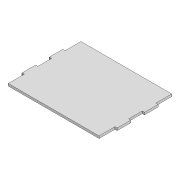
# Autodesk Inventor part: Tapa diagonal
Saved by Autodesk Inventor 2022 (Build 260153000, 153)
## iProperties
Created: 2022-06-16
Part Number: Tapa diagonal
Material: Generic
Document SubType Name: Modeling
Designer: ADMIN
Density: 1 g/cm^3
Appearance: Default
Author: ADMIN
Autodesk Inventor part; units mm, degrees
ref_plane "YZ Plane" through (0, 0, 0) normal (1, 0, 0) x (0, 1, 0)
ref_plane "XZ Plane" through (0, 0, 0) normal (0, 1, 0) x (-1, 0, 0)
ref_plane "XY Plane" through (0, 0, 0) normal (0, 0, 1) x (1, 0, 0)
sketch "Sketch1" plane through (0, 0, 0) normal (0, 1, 0) x (-1, 0, 0)
  line L0 (-88.7139, 28.3135) -> (111.2861, 28.3135)
  line L1 (111.2861, 28.3135) -> (111.2861, -131.6865)
  line L2 (111.2861, -131.6865) -> (-88.7139, -131.6865)
  line L3 (-88.7139, -131.6865) -> (-88.7139, 28.3135)
  line L4 (111.2861, -6.6865) -> (116.2861, -6.6865)
  line L5 (116.2861, -6.6865) -> (116.2861, -36.6865)
  line L6 (116.2861, -36.6865) -> (111.2861, -36.6865)
  line L7 (111.2861, -36.6865) -> (111.2861, -6.6865)
  line L8 (111.2861, -66.6865) -> (116.2861, -66.6865)
  line L9 (116.2861, -66.6865) -> (116.2861, -96.6865)
  line L10 (116.2861, -96.6865) -> (111.2861, -96.6865)
  line L11 (111.2861, -96.6865) -> (111.2861, -66.6865)
  line L12 (111.2861, -51.6865) -> (-88.7139, -51.6865) construction
  line L13 (11.2861, 28.3135) -> (11.2861, -131.6865) construction
  line L14 (-88.7139, -6.6865) -> (-93.7139, -6.6865)
  line L15 (-93.7139, -6.6865) -> (-93.7139, -36.6865)
  line L16 (-93.7139, -36.6865) -> (-88.7139, -36.6865)
  line L17 (-88.7139, -66.6865) -> (-93.7139, -66.6865)
  line L18 (-93.7139, -66.6865) -> (-93.7139, -96.6865)
  line L19 (-93.7139, -96.6865) -> (-88.7139, -96.6865)
  line L20 (-88.7139, -51.6865) -> (111.2861, -51.6865) construction
  point P0 (0, 0)
  dimension "d0" = 200
  dimension "d1" = 160
  dimension "d2" = 5
  dimension "d3" = 30
  dimension "d4" = 5
  dimension "d5" = 30
  dimension "d6" = 30
  dimension "d7" = 15
  constraints: 42 end point, 10 symmetric about line, 6 parallel, 4 midpoint, 3 horizontal, 3 perpendicular, 2 point on line
  measures "d0" distance of L1.end L2.end
  measures "d1" distance of L0.end L1.end
  measures "d2" distance of L5.end L6.end
  measures "d3" distance of L4.end L5.end
  measures "d4" distance of L9.end L10.end
  measures "d5" distance of L8.end L9.end
  measures "d6" distance between parallel lines of L8 L6
  measures "d7" distance between parallel lines of L12 L6
extrude "Extrusion1" add sketch "Sketch1" along normal blind 5
body "Solid1"
